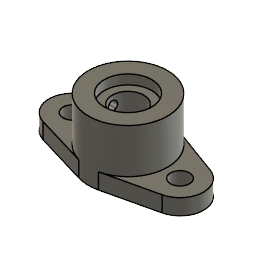
Record 7 (Autodesk Fusion 360 design; units mm, degrees)
part number: 2025-09-29-18-00-40-152
Autodesk Fusion 360 part; units mm, degrees
sketch "Sketch1" plane through (0, 0, 0) normal (0, 1, 0) x (1, 0, 0)
  circle A0 centre (0, 0) radius 25
  circle A1 centre (0, 0) radius 15
  circle A2 centre (0, 0) radius 10
  circle A3 centre (-35, 0) radius 6
  circle A4 centre (35, -2.1327) radius 6
  arc A5 (-39.2857, 14.3747) -> (-39.2857, -14.3747) centre (-35, 0) ccw
  arc A6 (38.3954, -16.7434) -> (40.1443, 11.9576) centre (35, -2.1327) ccw
  line L0 (8.5738, 23.4838) -> (40.1443, 11.9576)
  line L1 (5.659, -24.3511) -> (38.3954, -16.7434)
  line L2 (-39.2857, 14.3747) -> (-7.1429, 23.9579)
  line L3 (-7.1429, -23.9579) -> (-39.2857, -14.3747)
  arc A7 (8.5738, 23.4838) -> (-7.1429, 23.9579) centre (0, 0) ccw
  arc A8 (-7.1429, -23.9579) -> (5.659, -24.3511) centre (0, 0) ccw
  dimension "d3" = 50
  dimension "d4" = 30
  dimension "d5" = 20
  dimension "d8" = 12
  dimension "d9" = 12
  dimension "d10" = 35
  dimension "d11" = 35
  dimension "d12" = 30
  dimension "d13" = 30
  constraint coincident A0.centre A1.centre
  constraint concentric A3 A5
  constraint concentric A4 A6
  constraint coincident A0 L0.start
  constraint tangent A6 L0
  constraint coincident A0 L1.start
  constraint coincident A6 L1.end
  constraint coincident A5 L2.start
  constraint coincident A0 L2.end
  constraint coincident A0 L3.start
  constraint coincident A5 L3.end
  constraint coincident L1 A6.start
  constraint coincident L3 A5.end
  constraint coincident L2 A5.start
  constraint tangent A0 L2
  constraint tangent A0 L0
  constraint tangent A5 L2
  constraint tangent A5 L3
  constraint tangent A0 L3
  constraint tangent A0 L1
  constraint tangent A6 L1
  constraint tangent L2 A7
  constraint tangent L3 A8
  measures "d3" diameter of A0
  measures "d4" diameter of A1
  measures "d5" diameter of A2
  measures "d8" diameter of A3
  measures "d9" diameter of A4
  measures "d10" horizontal distance of A0.centre A4.centre
  measures "d11" distance of A0.centre A3.centre
  measures "d12" diameter of A5
  measures "d13" diameter of A6
extrude "Extrude1" add sketch "Sketch1" along normal blind 10 contours A0 A6 L0 L1 | A0 A5 L2 L3 makes body 1 at (-31.6163, 0, 10.1046) makes body 2 at (31.0948, 10, 12.0614)
sketch "Sketch2" plane through (0, 0, 0) normal (0, 1, 0) x (1, 0, 0)
  circle A0 centre (0, 0) radius 25
  circle A1 centre (0, 0) radius 15
  dimension "d16" = 50
  dimension "d17" = 30
  constraint coincident A0.centre A1.centre
  measures "d16" diameter of A0
  measures "d17" diameter of A1
extrude "Extrude2" add sketch "Sketch2" along normal blind 38 bodies 1 2
sketch "Sketch3" plane through (0, 0, 0) normal (0, 1, 0) x (1, 0, 0)
  circle A0 centre (0, 0) radius 15
  dimension "d20" = 30
  constraint coincident A0.centre origin
  measures "d20" diameter of A0
extrude "Extrude3" add sketch "Sketch3" along normal blind 38 bodies 1
sketch "Sketch4" plane through (0, 38, 0) normal (0, 1, 0) x (-1, 0, 0)
  circle A0 centre (0, 0) radius 25
  circle A1 centre (0, 0) radius 15
  circle A2 centre (0, 0) radius 10
  dimension "d23" = 30
  dimension "d24" = 20
  constraint coincident A0.centre A1.centre
  measures "d23" diameter of A1
  measures "d24" diameter of A2
extrude "Extrude4" cut sketch "Sketch4" along normal mid plane 12 contours A1 bodies 1
extrude "Extrude5" cut 1 faces at (2.7541, 38, -1.0148) along direction (0, 1, 0) mid plane 76 on bodies 1 bodies 1
sketch "Sketch5" plane through (0, 0, 0) normal (1, 0, 0) x (0, 0, -1)
  circle A0 centre (0, 26) radius 3
  point P0 (0, 38)
  dimension "d29" = 6
  dimension "d30" = 12
  measures "d29" diameter of A0
  measures "d30" distance of A0.centre P0
extrude "Extrude6" cut sketch "Sketch5" against normal blind 25 bodies 1
sketch "Sketch6" plane through (0, 0, 0) normal (1, 0, 0) x (0, 0, -1)
